Support Alim DCDC (Autodesk Fusion 360 design; units mm, degrees)
Autodesk Fusion 360 part; units mm, degrees
note: some values were not read from the file. Set by a fixed rule: which sketch regions a step uses.
sketch "Sketch1" plane through (0, 0, 0) normal (0, 0, 1) x (1, 0, 0)
  line L0 (21.5, -33.5) -> (-21.5, -33.5)
  line L1 (-25, -30) -> (-25, 30)
  line L2 (-21.5, 33.5) -> (21.5, 33.5)
  line L3 (25, 30) -> (25, -30)
  line L4 (25, -33.5) -> (-25, 33.5) construction
  line L5 (-25, -33.5) -> (25, 33.5) construction
  line L6 (20.5, -29) -> (-20.5, -29) construction
  line L7 (-20.5, -29) -> (-20.5, 29) construction
  line L8 (-20.5, 29) -> (20.5, 29) construction
  line L9 (20.5, 29) -> (20.5, -29) construction
  line L10 (20.5, -29) -> (-20.5, 29) construction
  line L11 (-20.5, -29) -> (20.5, 29) construction
  circle A0 centre (-20.5, 29) radius 3.5
  circle A1 centre (20.5, 29) radius 3.5
  circle A2 centre (-20.5, -29) radius 3.5
  circle A3 centre (20.5, -29) radius 3.5
  circle A4 centre (-20.5, 29) radius 1.6
  circle A5 centre (20.5, 29) radius 1.6
  circle A6 centre (20.5, -29) radius 1.6
  circle A7 centre (-20.5, -29) radius 1.6
  arc A8 (-21.5, 33.5) -> (-25, 30) centre (-21.5, 30) ccw
  arc A9 (25, 30) -> (21.5, 33.5) centre (21.5, 30) ccw
  arc A10 (21.5, -33.5) -> (25, -30) centre (21.5, -30) ccw
  arc A11 (-25, -30) -> (-21.5, -33.5) centre (-21.5, -30) ccw
  line L12 (10, -27.5) -> (-10, -27.5) construction
  line L13 (-10, -27.5) -> (-10, 27.5) construction
  line L14 (-10, 27.5) -> (10, 27.5) construction
  line L15 (10, 27.5) -> (10, -27.5) construction
  line L16 (10, -27.5) -> (-10, 27.5) construction
  line L17 (-10, -27.5) -> (10, 27.5) construction
  circle A12 centre (-10, 27.5) radius 1.6
  circle A13 centre (10, 27.5) radius 1.6
  circle A14 centre (-10, -27.5) radius 1.6
  circle A15 centre (10, -27.5) radius 1.6
  line L18 (0, 33.5) -> (0, -33.5) construction
  dimension "d1" = 50
  dimension "d2" = 67
  dimension "d3" = 41
  dimension "d4" = 58
  dimension "d5" = 7
  dimension "d6" = 7
  dimension "d7" = 7
  dimension "d8" = 7
  dimension "d9" = 3.2
  dimension "d10" = 3.2
  dimension "d11" = 3.2
  dimension "d12" = 3.2
  dimension "d13" = 3.5
  dimension "d14" = 20
  dimension "d15" = 55
  dimension "d16" = 3.2
  dimension "d18" = 3.2
  dimension "d19" = 3.2
  dimension "d21" = 3.2
  constraint horizontal L0
  constraint perpendicular L0 L1
  constraint parallel L0 L2
  constraint parallel L1 L3
  constraint coincident L4 origin
  constraint coincident L5 origin
  constraint horizontal L6
  constraint perpendicular L6 L7
  constraint parallel L6 L8
  constraint parallel L7 L9
  constraint coincident L10 origin
  constraint coincident L11 origin
  constraint coincident L7.end L8.start
  constraint coincident L8.end L9.start
  constraint coincident L6.end L7.start
  constraint coincident L6.start L9.end
  constraint concentric A0 A4
  constraint concentric A3 A6
  constraint concentric A2 A7
  constraint coincident L4.end L2
  constraint coincident L4.end L1
  constraint tangent L2 A8
  constraint tangent L1 A8
  constraint coincident L5.end L2
  constraint coincident L5.end L3
  constraint tangent L2 A9
  constraint tangent L3 A9
  constraint equal A8 A9
  constraint coincident L4.start L3
  constraint coincident L4.start L0
  constraint tangent L3 A10
  constraint tangent L0 A10
  constraint equal A8 A10
  constraint coincident L5.start L0
  constraint coincident L5.start L1
  constraint tangent L0 A11
  constraint tangent L1 A11
  constraint equal A8 A11
  constraint horizontal L12
  constraint perpendicular L12 L13
  constraint parallel L12 L14
  constraint parallel L13 L15
  constraint coincident L16 origin
  constraint coincident L17 origin
  constraint coincident L13.end L14.start
  constraint coincident L14.end L15.start
  constraint coincident L12.end L13.start
  constraint coincident L12.start L15.end
  constraint vertical L18
  constraint midpoint L18 origin
  constraint coincident L2 L18.start
  measures "d1" distance of L4.end L5.end
  measures "d2" distance of L5.start L4.end
  measures "d3" distance of L7.end L8.end
  measures "d4" distance of L6.end L7.end
  measures "d5" diameter of A0
  measures "d6" diameter of A1
  measures "d7" diameter of A2
  measures "d8" diameter of A3
  measures "d9" diameter of A4
  measures "d10" diameter of A5
  measures "d11" diameter of A6
  measures "d12" diameter of A7
  measures "d13" radius of A8
  measures "d14" distance of L13.end L14.end
  measures "d15" distance of L12.end L13.end
  measures "d16" diameter of A12
  measures "d18" diameter of A13
  measures "d19" diameter of A14
  measures "d21" diameter of A15
extrude "Extrude1" add sketch "Sketch1" against normal blind 3 contours L0 L1 L2 L3 A8 A9 A10 A11 | A0 | A1 | A2 | A3
extrude "Extrude2" add sketch "Sketch1" along normal blind 10 contours A0 | A1 | A2 | A3
sketch "Sketch2" plane through (0, 0, -3) normal (0, 0, -1) x (1, 0, 0)
  circle A0 centre (-20.5, 29) radius 1.6
  circle A1 centre (-20.5, -29) radius 1.6
  circle A2 centre (10, 27.5) radius 1.6
  circle A3 centre (-10, -27.5) radius 1.6
  circle A4 centre (-10, 27.5) radius 1.6
  circle A5 centre (10, -27.5) radius 1.6
  arc A6 (-25, -30) -> (-21.5, -33.5) centre (-20.5, -29) ccw
  line L0 (-21.5, -33.5) -> (21.5, -33.5)
  arc A7 (21.5, -33.5) -> (25, -30) centre (21.5, -30) ccw
  line L1 (25, -30) -> (25, 30)
  arc A8 (25, 30) -> (21.5, 33.5) centre (21.5, 30) ccw
  line L2 (21.5, 33.5) -> (-21.5, 33.5)
  arc A9 (-21.5, 33.5) -> (-25, 30) centre (-20.5, 29) ccw
  line L3 (-25, 30) -> (-25, -30)
  circle A10 centre (-20.5, 29) radius 3
  circle A11 centre (-20.5, -29) radius 3
  circle A12 centre (20.5, 29) radius 3
  circle A13 centre (20.5, -29) radius 3
  point P0 (-21.5, -30)
  point P1 (-21.5, 30)
  point P2 (20.5, -29)
  point P3 (20.5, 29)
  point P4 (-21.5, -30)
  point P5 (-21.5, 30)
  point P6 (20.5, -29)
  point P7 (20.5, 29)
  point P8 (-21.5, -30)
  point P9 (-21.5, 30)
  dimension "d33" = 6
  dimension "d35" = 6
  dimension "d40" = 6
  dimension "d41" = 6
  constraint concentric A0 A10
  constraint concentric A1 A11
  constraint coincident P7 P3
  constraint coincident P6 P2
  measures "d33" diameter of A10
  measures "d35" diameter of A11
  measures "d40" diameter of A12
  measures "d41" diameter of A13
extrude "Extrude3" cut sketch "Sketch2" against normal blind 2.5 contours A10 | A11 | A12 | A13
fillet "Fillet2" radius 3.5 4 edges at (-23.7631, -27.7343, 0) (-23.7631, 30.2657, 0) (17.2369, 30.2657, 0) (17.2369, -27.7343, 0)
